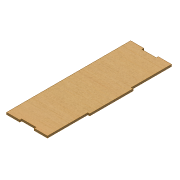
# Autodesk Inventor part: стенка 2
Saved by Autodesk Inventor 2021 (Build 250183000, 183)
## iProperties
Created: 2023-02-14
Part Number: стенка 2
Material: Типовые
Document SubType Name: Modeling
Designer: Tasya
Density: 1 g/cm^3
Appearance: Желтая сосна — массив — светлое морение — со слабым глянцем
Author: Tasya
Autodesk Inventor part; units mm, degrees
ref_plane "YZ Plane" through (0, 0, 0) normal (1, 0, 0) x (0, 1, 0)
ref_plane "XZ Plane" through (0, 0, 0) normal (0, 1, 0) x (-1, 0, 0)
ref_plane "XY Plane" through (0, 0, 0) normal (0, 0, 1) x (1, 0, 0)
sketch "Эскиз1" plane through (0, 0, 0) normal (0, 1, 0) x (-1, 0, 0)
  line L0 (-42.5, 129) -> (42.5, 129)
  line L1 (42.5, 129) -> (42.5, -129)
  line L2 (42.5, -129) -> (-42.5, -129)
  line L3 (-42.5, -129) -> (-42.5, 129)
  line L4 (-42.5, 129) -> (42.5, -129) construction
  line L5 (42.5, 129) -> (-42.5, -129) construction
  line L6 (0, 0) -> (-44.5, 0) construction
  line L7 (-42.5, 45) -> (-46.5, 45)
  line L8 (-46.5, 45) -> (-46.5, -45)
  line L9 (-46.5, -45) -> (-42.5, -45)
  line L10 (-42.5, -45) -> (-42.5, 45)
  line L11 (-42.5, 45) -> (-46.5, -45) construction
  line L12 (-46.5, 45) -> (-42.5, -45) construction
  line L13 (-15, 125) -> (15, 125)
  line L14 (15, 125) -> (15, 129)
  line L15 (15, 129) -> (-15, 129)
  line L16 (-15, 129) -> (-15, 125)
  line L17 (-15, 125) -> (15, 129) construction
  line L18 (15, 125) -> (-15, 129) construction
  line L19 (0, -163.7504) -> (0, 0) construction
  line L20 (-15, -125) -> (15, -125)
  line L21 (15, -125) -> (15, -129)
  line L22 (-15, -129) -> (-15, -125)
  line L23 (15, -129) -> (-15, -129)
  point P0 (0, 0)
  point P1 (-10, -165.5)
  point P2 (-10, -255.5)
  point P3 (-44.5, 0)
  point P4 (-10, -45)
  point P5 (-10, 45)
  point P6 (0, 127)
  point P7 (-5, -342)
  point P8 (5, -342)
  point P9 (5, 342)
  point P10 (-5, 342)
  point P11 (0, 0)
  point P12 (-42.5, 45)
  point P13 (-42.5, -45)
  point P14 (-15, -129)
  point P15 (15, -129)
  dimension "d0" = 258
  dimension "d1" = 85
  dimension "d5" = 90
  dimension "d6" = 4
  dimension "d7" = 4
  dimension "d8" = 30
  constraints: 48 end point, 8 midpoint, 6 parallel, 4 horizontal, 4 symmetric about line, 3 perpendicular, 2 collinear, 1 coincident, 1 vertical, 1 other
  measures "d0" distance of L2.end L0.start
  measures "d1" distance between parallel lines of L3 L1
  measures "d5" distance of L7.end L8.end
  measures "d6" distance of L8.end L9.end
  measures "d7" distance of L15.end L13.start
  measures "d8" distance of L13.start L13.end
extrude "Выдавливание1" add sketch "Эскиз1" along normal blind 4 contours L0 L16 L13 L14 L1 L2 L21 L20 L22 L3 | L3 L9 L8 L7
